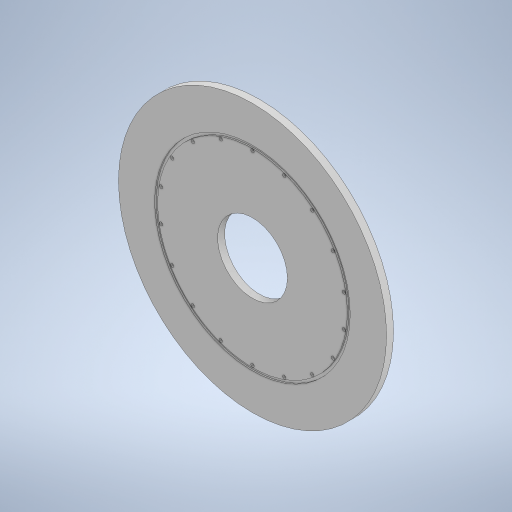
# Autodesk Inventor part: Brida_2 (flange_2) Lebus
Saved by Autodesk Inventor 2024.3 (Build 283343000, 343)
## iProperties
Created: 2025-07-02
Part Number: Brida_2 (flange_2) Lebus
Material: Genérico
Document SubType Name: Modeling
Designer: Daniel Rodriguez
Density: 1 g/cm^3
Appearance: Valor por defecto
Author: Daniel Rodriguez
Autodesk Inventor part; units mm, degrees
ref_plane "YZ Plane" through (0, 0, 0) normal (1, 0, 0) x (0, 1, 0)
ref_plane "XZ Plane" through (0, 0, 0) normal (0, 1, 0) x (-1, 0, 0)
ref_plane "XY Plane" through (0, 0, 0) normal (0, 0, 1) x (1, 0, 0)
sketch "Boceto1" plane through (0, 0, 0) normal (0, 0, 1) x (1, 0, 0)
  circle A0 centre (0, 0) radius 125
  circle A1 centre (0, 0) radius 480
  dimension "d0" = 960
  dimension "d1" = 250
  constraints: 2 centre point, 2 coincident
  measures "d0" diameter of A1
  measures "d1" diameter of A0
extrude "Extrusión1" add sketch "Boceto1" against normal blind 25
sketch "Boceto2" plane through (0, 0, 0) normal (0, 0, 1) x (1, 0, 0)
  circle A0 centre (0, 0) radius 350
  circle A1 centre (0, 0) radius 340
  dimension "d4" = 700
  dimension "d5" = 680
  constraints: 2 centre point, 2 coincident
  measures "d4" diameter of A0
  measures "d5" diameter of A1
extrude "Extrusión2" cut sketch "Boceto2" against normal blind 5
sketch "Boceto3" plane through (0, 0, 0) normal (0, 0, 1) x (1, 0, 0)
  circle A0 centre (0, 0) radius 332.5 construction
  circle A1 centre (0, 332.5) radius 6
  circle A2 centre (-113.7217, 312.4478) radius 6
  circle A3 centre (-213.7269, 254.7098) radius 6
  circle A4 centre (-287.9534, 166.25) radius 6
  circle A5 centre (-327.4486, 57.738) radius 6
  circle A6 centre (-327.4486, -57.738) radius 6
  circle A7 centre (-287.9534, -166.25) radius 6
  circle A8 centre (-213.7269, -254.7098) radius 6
  circle A9 centre (-113.7217, -312.4478) radius 6
  circle A10 centre (0, -332.5) radius 6
  circle A11 centre (113.7217, -312.4478) radius 6
  circle A12 centre (213.7269, -254.7098) radius 6
  circle A13 centre (287.9534, -166.25) radius 6
  circle A14 centre (327.4486, -57.738) radius 6
  circle A15 centre (327.4486, 57.738) radius 6
  circle A16 centre (287.9534, 166.25) radius 6
  circle A17 centre (213.7269, 254.7098) radius 6
  circle A18 centre (113.7217, 312.4478) radius 6
  dimension "d8" = 665
  dimension "d9" = 12
  dimension "d12" = 360
  constraints: 18 centre point, 1 coincident, 1 vertical alignment, 39 other
  measures "d9" diameter of A1
extrude "Extrusión3" cut sketch "Boceto3" against normal up to next
